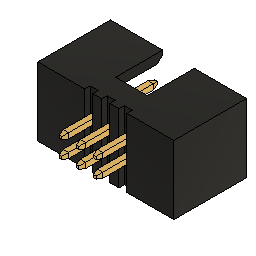
IDC_1.27mm (Autodesk Fusion 360 design; units mm, degrees)
Autodesk Fusion 360 part; units mm, degrees
sketch "Sketch1" plane through (0, 0, 0) normal (0, 1, 0) x (1, 0, 0)
  line L0 (5.055, -2.55) -> (-5.055, -2.55)
  line L1 (-5.055, -2.55) -> (-5.055, 2.55)
  line L2 (-5.055, 2.55) -> (5.055, 2.55)
  line L3 (5.055, 2.55) -> (5.055, -2.55)
  line L4 (5.055, 2.55) -> (-5.055, -2.55) construction
  dimension "d2" = 5.1
  dimension "d3" = 10.11
  constraint horizontal L0
  constraint vertical L1
  constraint horizontal L2
  constraint vertical L3
  constraint midpoint origin L4
  measures "d2" distance of L0.start L2.end
  measures "d3" distance of L0.start L0.end
extrude "Extrude1" add sketch "Sketch1" along normal blind 1.9 makes body 1
sketch "Sketch2" plane through (0, 1.9, 0) normal (0, 1, 0) x (-1, 0, 0)
  line L0 (-5.055, -2.55) -> (5.055, -2.55)
  line L1 (5.055, -2.55) -> (5.055, 2.55)
  line L2 (5.055, 2.55) -> (-5.055, 2.55)
  line L3 (-5.055, 2.55) -> (-5.055, -2.55)
  line L4 (-4.355, 1.85) -> (4.355, 1.85)
  line L5 (4.355, 1.85) -> (4.355, -1.85)
  line L6 (4.355, -1.85) -> (-4.355, -1.85)
  line L7 (-4.355, -1.85) -> (-4.355, 1.85)
  line L8 (-1.175, 1.85) -> (1.175, 1.85)
  line L9 (1.175, 1.85) -> (1.175, 2.55)
  line L10 (1.175, 2.55) -> (-1.175, 2.55)
  line L11 (-1.175, 2.55) -> (-1.175, 1.85)
  point P0 (0, 2.55)
  dimension "d6" = 0.7
  dimension "d7" = 0.7
  dimension "d8" = 0.7
  dimension "d9" = 0.7
  dimension "d10" = 2.35
  constraint horizontal L4
  constraint vertical L5
  constraint horizontal L6
  constraint vertical L7
  constraint horizontal L8
  constraint vertical L9
  constraint horizontal L10
  constraint vertical L11
  constraint coincident L2 L9.end
  constraint coincident L4 L8.start
  constraint midpoint L2 P0
  constraint midpoint L10 P0
  measures "d6" distance of L3 L7
  measures "d7" distance of L0 L6
  measures "d8" distance of L1 L5
  measures "d9" distance of L2 L4
  measures "d10" distance of L9.end L10.end
extrude "Extrude2" add sketch "Sketch2" along normal blind 3.5 contours L0 L1 L2 L3 L4 L5 L6 L7 L9 L11 bodies 1
chamfer "Chamfer1" distance 0.4 angle 45 5 edges at (-2.765, 5.4, 1.85) (-4.355, 5.4, 0) (0, 5.4, -1.85) (4.355, 5.4, 0) (2.765, 5.4, 1.85) on bodies 1
sketch "Sketch3" plane through (0, 0, 0) normal (0, -1, 0) x (1, 0, 0)
  line L0 (-5.055, -2.55) -> (5.055, -2.55)
  line L1 (5.055, -2.55) -> (5.055, 2.55)
  line L2 (5.055, 2.55) -> (-5.055, 2.55)
  line L3 (-5.055, 2.55) -> (-5.055, -2.55)
  line L4 (1.57, -2.55) -> (1.57, 2.55)
  line L5 (0.97, -2.55) -> (0.97, 2.55)
  line L6 (1.47, -0.835) -> (1.07, -0.835)
  line L7 (1.07, -0.835) -> (1.07, -0.435)
  line L8 (1.07, -0.435) -> (1.47, -0.435)
  line L9 (1.47, -0.435) -> (1.47, -0.835)
  line L10 (1.47, 0.435) -> (1.07, 0.435)
  line L11 (1.07, 0.435) -> (1.07, 0.835)
  line L12 (1.07, 0.835) -> (1.47, 0.835)
  line L13 (1.47, 0.835) -> (1.47, 0.435)
  dimension "d14" = 0.6
  dimension "d15" = 3.485
  dimension "d26" = 0.1
  dimension "d27" = 0.4
  dimension "d28" = 1.715
  dimension "d29" = 0.87
  constraint coincident L0 L4.start
  constraint coincident L2 L4.end
  constraint perpendicular L2 L4
  constraint coincident L0 L5.start
  constraint coincident L2 L5.end
  constraint perpendicular L2 L5
  constraint horizontal L6
  constraint vertical L7
  constraint horizontal L8
  constraint vertical L9
  constraint horizontal L10
  constraint vertical L11
  constraint horizontal L12
  constraint vertical L13
  constraint equal L6 L9
  constraint equal L10 L13
  constraint vertical L8.end L10.start
  constraint vertical L7.end L10.end
  measures "d14" distance of L4.start L5.start
  measures "d15" distance of L0.end L4.start
  measures "d26" distance of L4 L6.start
  measures "d27" distance of L6.start L6.end
  measures "d28" vertical distance of L4.start L6.start
  measures "d29" distance of L8.end L10.start
extrude "Extrude3" cut sketch "Sketch3" against normal blind 0.4 contours L0 L2 L4 L5 | L6 L7 L8 L9 | L10 L11 L12 L13 bodies 1
extrude "Extrude4" cut sketch "Sketch3" against normal blind 1.9 contours L6 L7 L8 L9 | L10 L11 L12 L13 bodies 1
pattern_linear "R-Pattern1" count 3 spacing 1.27 along (-1, 0, 0) of "Extrude3", "Extrude4"
ref_plane "WorkPlane1" through (0, -2.1, 0) normal (0, -1, 0) x (-1, 0, 0)
sketch "Sketch5" plane through (0, -2.1, 0) normal (0, -1, 0) x (-1, 0, 0)
  line L0 (-1.07, -0.835) -> (-1.47, -0.835)
  line L1 (-1.47, -0.835) -> (-1.47, -0.435)
  line L2 (-1.47, -0.435) -> (-1.07, -0.435)
  line L3 (-1.07, -0.435) -> (-1.07, -0.835)
extrude "Extrude5" add sketch "Sketch5" against normal blind 7.1 separate body makes body 2
chamfer "Chamfer2" distance 0.4 distance2 0.1 4 edges at (1.27, -2.1, 0.435) (1.27, -2.1, 0.835) (1.47, -2.1, 0.635) (1.07, -2.1, 0.635) measured on face at (1.3367, 0.2667, 0.435) measured on face at (1.2033, 0.2667, 0.835) measured on face at (1.47, 0.2667, 0.7017) measured on face at (1.07, 0.2667, 0.5683) on bodies 2
chamfer "Chamfer2" distance 0.1 distance2 0.4 4 edges at (1.27, 5, 0.435) (1.07, 5, 0.635) (1.27, 5, 0.835) (1.47, 5, 0.635) measured on face at (1.2033, 5, 0.7017) measured on face at (1.2033, 5, 0.7017) measured on face at (1.2033, 5, 0.7017) measured on face at (1.2033, 5, 0.7017) on bodies 2
pattern_linear "R-Pattern2" count 3 spacing 1.27 along (-1, 0, 0) count 2 spacing 1.27 along (0, 0, -1) of bodies 2 makes body 3 at (-0.0667, 0.4, 0.835) makes body 4 at (1.2033, 0.4, -0.435) makes body 5 at (-0.0667, 0.4, -0.435) makes body 6 at (-1.3367, 0.4, 0.835) makes body 7 at (-1.3367, 0.4, -0.435)
equation "row_size = 3"
equation "d3 = 3.585 mm * 2 + 0.4 mm + ( 1.27 * ( row_size - 1 ) ) * 1 mm"
equation "d22 = row_size"
equation "d24 = 0.6 mm + 0.67 mm"
equation "d39 = row_size"
